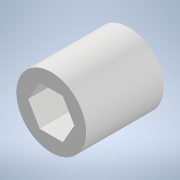
# Autodesk Inventor part: tubo
Saved by Autodesk Inventor 2020.3 (Build 243373000, 373)
## iProperties
Created: 2021-02-02
Part Number: tubo
Material: Generic
Document SubType Name: Modeling
Designer: Yu Jinyu
Density: 1 g/cm^3
Appearance: Default
Author: Yu Jinyu
Autodesk Inventor part; units mm, degrees
ref_plane "YZ Plane" through (0, 0, 0) normal (1, 0, 0) x (0, 1, 0)
ref_plane "XZ Plane" through (0, 0, 0) normal (0, 1, 0) x (-1, 0, 0)
ref_plane "XY Plane" through (0, 0, 0) normal (0, 0, 1) x (1, 0, 0)
sketch "Sketch1" plane through (0, 0, 0) normal (0, 0, 1) x (1, 0, 0)
  circle A0 centre (0, 0) radius 11.25
  dimension "d0" = 22.5
  constraints: 1 centre point, 1 coincident
  measures "d0" diameter of A0
extrude "Extrusion1" add sketch "Sketch1" along normal blind 25
sketch "Sketch2" plane through (0, 0, 0) normal (0, 0, -1) x (-1, 0, 0)
  line L0 (7.6788, 0) -> (3.8394, -6.65)
  line L1 (3.8394, -6.65) -> (-3.8394, -6.65)
  line L2 (-3.8394, -6.65) -> (-7.6788, 0)
  line L3 (-7.6788, 0) -> (-3.8394, 6.65)
  line L4 (-3.8394, 6.65) -> (3.8394, 6.65)
  line L5 (3.8394, 6.65) -> (7.6788, 0)
  point P0 (0, 0)
  point P1 (0, 0)
  dimension "d3" = 13.3
  constraints: 12 end point, 1 coincident, 13 other
  measures "d3" distance between parallel lines of L2 L5
extrude "Extrusion2" cut sketch "Sketch2" against normal blind 30
sketch "Sketch3" plane through (0, 0, 25) normal (0, 0, 1) x (1, 0, 0)
  line L0 (3.8394, 6.65) -> (7.6788, 0) projected
  line L1 (7.6788, 0) -> (3.8394, -6.65) projected
  line L2 (3.8394, -6.65) -> (-3.8394, -6.65) projected
  line L3 (-3.8394, -6.65) -> (-7.6788, 0) projected
  line L4 (-7.6788, 0) -> (-3.8394, 6.65) projected
  line L5 (-3.8394, 6.65) -> (3.8394, 6.65) projected
  circle A0 centre (0, 0) radius 11.25 projected
extrude "Extrusion3" add sketch "Sketch3" along normal blind 10
body "Solid1"
